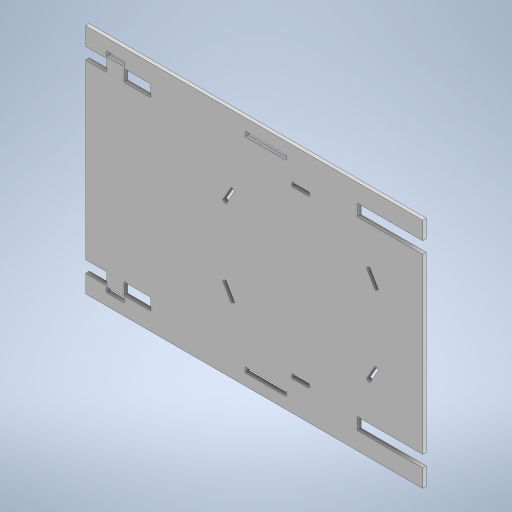
# Autodesk Inventor part: base_ver2
Saved by Autodesk Inventor 2024 (Build 280153000, 153)
## iProperties
Created: 2024-03-29
Part Number: base_ver2
Material: Generic
Document SubType Name: Modeling
Designer: op04o
Density: 1 g/cm^3
Appearance: Default
Author: op04o
Autodesk Inventor part; units mm, degrees
ref_plane "YZ Plane" through (0, 0, 0) normal (1, 0, 0) x (0, 1, 0)
ref_plane "XZ Plane" through (0, 0, 0) normal (0, 1, 0) x (-1, 0, 0)
ref_plane "XY Plane" through (0, 0, 0) normal (0, 0, 1) x (1, 0, 0)
sketch "Sketch1" plane through (0, 0, 0) normal (0, 0, 1) x (1, 0, 0)
  line L0 (0.909, 16.8369) -> (0.909, 1.3644)
  line L1 (0.909, 1.3644) -> (290.909, 1.3644)
  line L2 (0.909, 175.8919) -> (0.909, 26.8369)
  line L3 (290.909, 185.9921) -> (290.909, 201.3644)
  line L4 (290.909, 201.3644) -> (0.909, 201.3644)
  line L5 (0.909, 201.3644) -> (0.909, 185.8919)
  line L6 (290.909, 26.7367) -> (290.909, 175.9921)
  line L7 (290.909, 1.3644) -> (290.909, 16.7367)
  line L8 (290.909, 26.7367) -> (290.909, 175.9921)
  line L9 (0.909, 16.8369) -> (0.909, 1.3644)
  line L10 (0.909, 1.3644) -> (290.909, 1.3644)
  line L11 (290.909, 1.3644) -> (290.909, 16.7367)
  line L12 (0.909, 175.8919) -> (0.909, 26.8369)
  line L13 (138.409, 187.457) -> (138.409, 191.457)
  line L14 (138.409, 191.457) -> (173.409, 191.457)
  line L15 (173.409, 191.457) -> (173.409, 187.457)
  line L16 (173.409, 187.457) -> (138.409, 187.457)
  line L17 (173.409, 11.457) -> (138.409, 11.457)
  line L18 (138.409, 11.457) -> (138.409, 15.457)
  line L19 (138.409, 15.457) -> (173.409, 15.457)
  line L20 (173.409, 15.457) -> (173.409, 11.457)
  line L21 (290.909, 175.9921) -> (234.909, 175.9921)
  line L22 (234.909, 175.9921) -> (234.909, 185.9921)
  line L23 (234.909, 185.9921) -> (290.909, 185.9921)
  line L24 (56.909, 185.8919) -> (56.909, 175.8919)
  line L25 (178.409, 173.457) -> (193.409, 173.457)
  line L26 (193.409, 173.457) -> (193.409, 170.457)
  line L27 (193.409, 170.457) -> (178.409, 170.457)
  line L28 (178.409, 170.457) -> (178.409, 173.457)
  line L29 (126.4391, 143.4522) -> (129.0372, 141.9522)
  line L30 (252.8788, 70.4522) -> (245.3788, 57.4618)
  line L31 (245.3788, 57.4618) -> (242.7807, 58.9618)
  line L32 (242.7807, 58.9618) -> (250.2807, 71.9522)
  line L33 (250.2807, 71.9522) -> (252.8788, 70.4522)
  line L34 (129.0372, 58.9618) -> (126.4391, 57.4618)
  line L35 (242.7807, 141.9522) -> (245.3788, 143.4522)
  line L36 (245.3788, 143.4522) -> (252.8788, 130.4618)
  line L37 (252.8788, 130.4618) -> (250.2807, 128.9618)
  line L38 (250.2807, 128.9618) -> (242.7807, 141.9522)
  line L39 (193.409, 27.457) -> (178.409, 27.457)
  line L40 (178.409, 27.457) -> (178.409, 30.457)
  line L41 (178.409, 30.457) -> (193.409, 30.457)
  line L42 (193.409, 30.457) -> (193.409, 27.457)
  line L43 (290.909, 26.7367) -> (234.909, 26.7367)
  line L44 (234.909, 26.7367) -> (234.909, 16.7367)
  line L45 (234.909, 16.7367) -> (290.909, 16.7367)
  line L46 (56.909, 16.8369) -> (56.909, 26.8369)
  line L47 (18.917, 187.457) -> (33.917, 187.457)
  line L48 (33.917, 187.457) -> (33.917, 191.457)
  line L49 (33.917, 191.457) -> (18.917, 191.457)
  line L50 (18.917, 191.457) -> (18.917, 187.457)
  line L51 (33.917, 11.457) -> (33.917, 15.457)
  line L52 (33.917, 15.457) -> (18.917, 15.457)
  line L53 (18.917, 15.457) -> (18.917, 11.457)
  line L54 (18.917, 11.457) -> (33.917, 11.457)
  line L55 (18.917, 185.8919) -> (18.917, 175.8919)
  line L56 (33.917, 185.8919) -> (33.917, 175.8919)
  line L57 (0.909, 185.8919) -> (18.917, 185.8919)
  line L58 (33.917, 185.8919) -> (56.909, 185.8919)
  line L59 (56.909, 175.8919) -> (33.917, 175.8919)
  line L60 (18.917, 175.8919) -> (0.909, 175.8919)
  line L61 (18.917, 26.8369) -> (18.917, 16.8369)
  line L62 (33.917, 16.8369) -> (33.917, 26.8369)
  line L63 (56.909, 26.8369) -> (33.917, 26.8369)
  line L64 (18.917, 26.8369) -> (0.909, 26.8369)
  line L65 (0.909, 16.8369) -> (18.917, 16.8369)
  line L66 (33.917, 16.8369) -> (56.909, 16.8369)
  line L67 (127.7381, 142.7022) -> (127.7381, 144.2022)
  line L68 (127.7381, 141.2022) -> (127.7381, 142.7022)
  line L69 (127.7381, 58.2118) -> (127.7381, 59.7118)
  line L70 (127.7381, 56.7118) -> (127.7381, 58.2118)
  line L71 (129.0372, 141.9522) -> (121.5372, 128.9618)
  line L72 (121.5372, 128.9618) -> (118.9391, 130.4618)
  line L73 (118.9391, 130.4618) -> (126.4391, 143.4522)
  line L74 (129.0372, 58.9618) -> (121.5372, 71.9522)
  line L75 (121.5372, 71.9522) -> (118.9391, 70.4522)
  line L76 (118.9391, 70.4522) -> (126.4391, 57.4618)
  dimension "d266" = 1.5
  dimension "d274" = 15
  dimension "d275" = 3
  dimension "d276" = 15
  dimension "d277" = 3
  constraints: 154 end point, 41 parallel, 10 perpendicular, 7 point on line, 2 midpoint, 2 vertical, 1 horizontal, 1 other
  measures "d266" distance of L69.start L69.end
  measures "d274" distance of L29.end L71.end
  measures "d275" distance of L71.end L72.end
  measures "d276" distance of L34.start L74.end
  measures "d277" distance of L74.end L75.end
extrude "Extrusion3" add sketch "Sketch1" along normal blind 3
body "Solid3"
